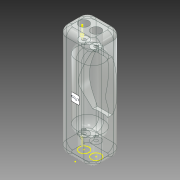
# Autodesk Inventor part: cable case standoff
Saved by Autodesk Inventor 2017 (Build 210142000, 142)
## iProperties
Created: 2018-09-03
Part Number: cable case standoff
Material: Steel
Document SubType Name: Modeling
Designer: ari
Density: 7.85 g/cm^3
Appearance: Clear
Mass: 84.9775 g
Surface Area: 67.7299 cm^2
Volume: 10.8252 cm^3
Author: ari
Autodesk Inventor part; units mm, degrees
ref_plane "YZ Plane" through (0, 0, 0) normal (1, 0, 0) x (0, 1, 0)
ref_plane "XZ Plane" through (0, 0, 0) normal (0, 1, 0) x (-1, 0, 0)
ref_plane "XY Plane" through (0, 0, 0) normal (0, 0, 1) x (1, 0, 0)
sketch "Sketch1" plane through (0, 0, 0) normal (0, 1, 0) x (-1, 0, 0)
  line L0 (-10, 31.5) -> (10, 31.5)
  line L1 (10, 31.5) -> (10, -31.5)
  line L2 (10, -31.5) -> (-10, -31.5)
  line L3 (-10, -31.5) -> (-10, 31.5)
  line L4 (-10, 31.5) -> (10, -31.5) construction
  line L5 (10, 31.5) -> (-10, -31.5) construction
  line L6 (0, 31.5) -> (0, -31.5) construction
  point P0 (0, 0)
  dimension "d0" = 20
  dimension "d1" = 63
  constraints: 14 end point, 4 midpoint, 2 parallel, 1 horizontal, 1 perpendicular
  measures "d0" distance of L0.start L0.end
  measures "d1" distance of L0.end L1.end
sketch "Sketch2" plane through (0, 0, 0) normal (0, 1, 0) x (-1, 0, 0)
  point P0 (0, 0)
extrude "Extrusion1" add sketch "Sketch1" along normal blind 17
sketch "Sketch3" plane through (0, 17, 0) normal (0, 1, 0) x (1, 0, 0)
  line L0 (-4, -14) -> (-11, 0) construction
  line L1 (-11, 0) -> (-4, 14) construction
  spline S0 degree 2 poles (-4, -14) (-11, 0) (-4, 14) knots 1 1 1 2 2 2 construction
  line L2 (7.5, -14) -> (-7.5, -14) construction
  line L3 (-7.5, -14) -> (-7.5, 14) construction
  line L4 (-7.5, 14) -> (7.5, 14) construction
  line L5 (7.5, 14) -> (7.5, -14) construction
  line L6 (7.5, -14) -> (-7.5, 14) construction
  line L7 (-7.5, -14) -> (7.5, 14) construction
  line L8 (-7.5, 0) -> (-11, 0) construction
  line L9 (0, 0) -> (0, 14) construction
  line L10 (4, -14) -> (11, 0) construction
  line L11 (11, 0) -> (4, 14) construction
  spline S1 degree 2 poles (4, -14) (11, 0) (4, 14) knots 1 1 1 2 2 2 construction
  line L12 (4, -14) -> (-4, -14) construction
  line L13 (4, 14) -> (-4, 14) construction
  line L14 (4.3102, -14.5) -> (11.5, 0) construction
  line L15 (11.5, 0) -> (4.3102, 14.5) construction
  spline S2 degree 2 poles (4.3102, -14.5) (11.5, 0) (4.3102, 14.5) knots 1 1 1 2 2 2
  line L16 (4.3102, -14.5) -> (-4.3102, -14.5)
  line L17 (4.3102, 14.5) -> (-4.3102, 14.5)
  line L18 (-4.3102, -14.5) -> (-11.5, 0) construction
  line L19 (-11.5, 0) -> (-4.3102, 14.5) construction
  spline S3 degree 2 poles (-4.3102, -14.5) (-11.5, 0) (-4.3102, 14.5) knots 1 1 1 2 2 2
  dimension "d4" = 3.5
  dimension "d5" = 28
  dimension "d6" = 15
  dimension "d20" = 0.5
  dimension "d21" = 0.5
  dimension "d22" = 0.5
  dimension "d23" = 8
  constraints: 24 end point, 6 symmetric about line, 4 midpoint, 3 parallel, 3 point on line, 2 collinear, 2 horizontal, 2 perpendicular, 1 coincident, 1 vertical, 14 other
  measures "d4" distance from line of L3 L0.end
  measures "d5" distance of L4.end L2.start
  measures "d6" distance of L3.end L4.end
  measures "d20" distance of L10.end L14.end
  measures "d21" distance between parallel lines of L16 L12
  measures "d22" distance from line of L11.end L15
  measures "d23" distance of L10.start L0.start
fillet "Fillet1" radius 5 4 edges at (-10, 17, 0) (-10, 0, 0) (10, 0, 0) (10, 17, 0)
sketch "Sketch4" plane through (5, 0, -31.5) normal (0, 0, -1) x (-1, 0, 0)
  arc A0 (0, 17) -> (-5, 12) centre (0, 12) ccw construction
  line L0 (-5, 5) -> (-5, 12) construction
  arc A1 (-5, 5) -> (0, 0) centre (0, 5) ccw construction
  line L1 (10, 0) -> (0, 0) construction
  arc A2 (10, 0) -> (15, 5) centre (10, 5) ccw construction
  line L2 (15, 5) -> (15, 12) construction
  arc A3 (15, 12) -> (10, 17) centre (10, 12) ccw construction
  line L3 (0, 17) -> (10, 17) construction
  line L4 (15, 5) -> (15, 12) construction
  line L5 (15, 8.5) -> (-5, 8.5) construction
  line L6 (5, 0) -> (5, 17) construction
  line L7 (0, 17) -> (10, 17) construction
  circle A4 centre (8.5, 8.5) radius 2.75
  line L8 (5.75, 8.5) -> (5.75, 0) construction
  dimension "d8" = 5.5
  dimension "d9" = 0.75
  constraints: 6 end point, 3 midpoint, 3 point on line, 1 horizontal alignment, 1 perpendicular, 2 other
  measures "d9" distance between parallel lines of L6 L8
extrude "Extrusion2" cut sketch "Sketch4" against normal blind 8
sketch "Sketch5" plane through (-3.5, 8.5, -23.5) normal (0, 0, -1) x (-1, 0, 0)
  circle A0 centre (0, 0) radius 2.75 projected
  circle A1 centre (0, 0) radius 1
  point P0 (-3.5, -8.5)
  dimension "d12" = 2
  constraints: 1 centre point, 1 coincident
  measures "d12" diameter of A1
extrude "Extrusion3" cut sketch "Sketch5" against normal blind 2 contours A1
mirror "Mirror1" about plane through (0, 0, 0) normal (1, 0, 0) of "Extrusion2", "Extrusion3"
mirror "Mirror2" about plane through (0, 0, 0) normal (0, 0, 1) of "Extrusion2", "Extrusion3", "Mirror1"
sketch "Sketch6" plane through (0, 0, 0) normal (0, 0, 1) x (1, 0, 0)
  line L0 (1.5, 8.5) -> (-1.5, 8.5) construction
  line L1 (1.5, 15) -> (-1.5, 15)
  line L2 (-1.5, 2) -> (1.5, 2)
  arc A0 (1.5, 2) -> (1.5, 15) centre (1.5, 8.5) ccw
  arc A1 (-1.5, 15) -> (-1.5, 2) centre (-1.5, 8.5) ccw
  line L3 (0, 18) -> (0, -3) construction
  circle A2 centre (3.5, 8.5) radius 1 construction
  point P0 (0, 8.5)
  dimension "d15" = 16
  dimension "d16" = 13
  constraints: 8 end point, 4 point on circle, 4 tangent, 2 centre point, 2 point on line, 1 horizontal, 1 midpoint, 1 parallel
  measures "d16" distance between parallel lines of L1 L2
extrude "Extrusion4" cut sketch "Sketch6" along normal up to surface (43 mm away) from surface at -21.5
fillet "Fillet2" radius 4 8 edges at (0, 2, 21.5) (-8, 8.5, 21.5) (0, 15, 21.5) (8, 8.5, 21.5) (8, 8.5, -21.5) (0, 15, -21.5) (-8, 8.5, -21.5) (0, 2, -21.5)
extrude "Extrusion5" cut sketch "Sketch3" against normal up to next
fillet "Fillet3" radius 3.5 16 edges at (8.5355, 15.5355, -31.5) (0, 17, -31.5) (-8.5355, 15.5355, -31.5) (-10, 8.5, -31.5) (-8.5355, 1.4645, -31.5) (0, 0, -31.5) (8.5355, 1.4645, -31.5) (10, 8.5, -31.5) (8.5355, 15.5355, 31.5) (0, 17, 31.5) (-8.5355, 15.5355, 31.5) (-10, 8.5, 31.5) (-8.5355, 1.4645, 31.5) (0, 0, 31.5) (8.5355, 1.4645, 31.5) (10, 8.5, 31.5)
sketch "Sketch7" plane through (5, 3.5, -31.5) normal (0, 0, -1) x (-1, 0, 0)
  circle A0 centre (1.5, 5) radius 2.75 projected
  circle A1 centre (8.5, 5) radius 2.75 projected
  point P0 (5, -3.5)
extrude "Extrusion6" [suppressed]
hole "Hole1" [suppressed]
mirror "Mirror3" [suppressed]
body "Solid1"
